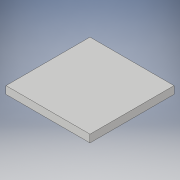
# Autodesk Inventor part: Peltier
Saved by Autodesk Inventor 2019 (Build 230136000, 136)
## iProperties
Created: 2019-01-30
Part Number: Peltier
Material: Ogólny
Document SubType Name: Modeling
Designer: atmat
Density: 1 g/cm^3
Appearance: Domyślna
Author: atmat
Autodesk Inventor part; units mm, degrees
ref_plane "YZ Plane" through (0, 0, 0) normal (1, 0, 0) x (0, 1, 0)
ref_plane "XZ Plane" through (0, 0, 0) normal (0, 1, 0) x (-1, 0, 0)
ref_plane "XY Plane" through (0, 0, 0) normal (0, 0, 1) x (1, 0, 0)
sketch "Szkic1" plane through (0, 0, 0) normal (0, 1, 0) x (-1, 0, 0)
  line L0 (20, 20) -> (-20, 20)
  line L1 (-20, 20) -> (-20, -20)
  line L2 (-20, -20) -> (20, -20)
  line L3 (20, -20) -> (20, 20)
  point P0 (0, 0)
  dimension "d0" = 40
  dimension "d1" = 40
  dimension "d2" = 20
  dimension "d3" = 20
  constraints: 8 end point, 2 parallel, 1 horizontal, 1 perpendicular
  measures "d0" distance of L2.end L0.start
  measures "d1" distance of L1.end L2.end
  measures "d2" distance from line of point (0, 0) L2
  measures "d3" distance from line of L3 point (0, 0)
extrude "Wyciągnięcie proste1" add sketch "Szkic1" along normal blind 3.6
